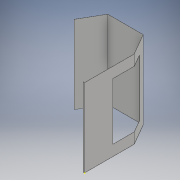
# Autodesk Inventor part: Cover 1
Saved by Autodesk Inventor 2018 (Build 220112000, 112)
## iProperties
Created: 2018-03-20
Part Number: Cover 1
Material: Generic
Document SubType Name: Modeling
Designer: p446024
Density: 1 g/cm^3
Appearance: Default
Author: p446024
Autodesk Inventor part; units mm, degrees
ref_plane "YZ Plane" through (0, 0, 0) normal (1, 0, 0) x (0, 1, 0)
ref_plane "XZ Plane" through (0, 0, 0) normal (0, 1, 0) x (-1, 0, 0)
ref_plane "XY Plane" through (0, 0, 0) normal (0, 0, 1) x (1, 0, 0)
sketch "Sketch1" plane through (0, 0, 0) normal (0, 0, 1) x (1, 0, 0)
  line L0 (0, 0) -> (20, 0)
  line L1 (20, 0) -> (20, 700)
  line L2 (20, 700) -> (-153, 999.6448)
  line L3 (-153, 999.6448) -> (-653, 999.6448)
  line L4 (-653, 999.6448) -> (-826, 700)
  line L5 (-824.1525, 700) -> (-652.0762, 998.0448)
  line L6 (-652.0762, 998.0448) -> (-153.9238, 998.0448)
  line L7 (-153.9238, 998.0448) -> (18.4, 699.5713)
  line L8 (18.4, 699.5713) -> (18.4, 1.6)
  line L9 (18.4, 1.6) -> (0, 1.6)
  line L10 (-826, 700) -> (-824.1525, 700)
  line L11 (0, 1.6) -> (0, 0)
  dimension "d0" = 20
  dimension "d1" = 700
  dimension "d2" = 90
  dimension "d3" = 346
  dimension "d4" = 150
  dimension "d5" = 500
  dimension "d6" = 346
  dimension "d7" = 120
  dimension "d8" = 1.6
  constraints: 24 end point, 3 horizontal, 2 perpendicular, 1 vertical, 4 other
  measures "d0" distance of L0.start L0.end
  measures "d1" distance of L0.end L1.end
  measures "d2" angle of L1 L0
  measures "d3" distance of L1.end L2.end
  measures "d4" angle of L2 L1
  measures "d5" distance of L2.end L3.end
  measures "d6" distance of L3.end L4.end
  measures "d7" angle of L4 L3
  measures "d8" distance between parallel lines of L2 L7
extrude "main" add sketch "Sketch1" along normal blind 1100
sketch "Sketch2" plane through (20, 0, 0) normal (1, 0, 0) x (0, 0, -1)
  point P0 (0, 0)
sketch "Sketch3" plane through (20, 0, 0) normal (1, 0, 0) x (0, 0, -1)
  line L0 (-1100, 0) -> (-1100, 700) projected
  line L1 (-950, 400) -> (-150, 400)
  line L2 (-150, 400) -> (-150, 700)
  line L3 (-150, 700) -> (-950, 700)
  line L4 (-950, 700) -> (-950, 400)
  line L5 (-950, 700) -> (-150, 700)
  point P0 (0, 0)
  dimension "d13" = 800
  dimension "d14" = 300
  constraints: 10 end point, 2 horizontal, 2 parallel, 1 perpendicular
  measures "d13" distance of L1.start L1.end
  measures "d14" distance of L1.end L2.end
sketch "Sketch4" plane through (-153, 999.6448, 1100) normal (0.866, 0.5, 0) x (0, 0, -1)
  line L0 (1100, -346) -> (0, -346) projected
  line L1 (151.2631, -346) -> (951.2631, -346)
  line L2 (951.2631, -346) -> (951.2631, -146)
  line L3 (951.2631, -146) -> (151.2631, -146)
  line L4 (151.2631, -146) -> (151.2631, -346)
  point P0 (1100, -942.2178)
  dimension "d16" = 800
  dimension "d17" = 200
  constraints: 8 end point, 2 parallel, 1 horizontal, 1 perpendicular, 1 point on line
  measures "d16" distance of L2.end L3.end
  measures "d17" distance of L1.end L2.end
extrude "Extrusion2" cut sketch "Sketch4" against normal blind 1.6
extrude "Extrusion3" cut sketch "Sketch3" against normal blind 1.6
body "Solid1"
